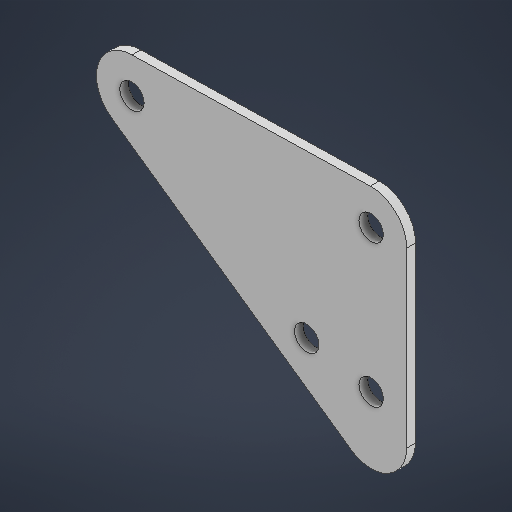
# Autodesk Inventor part: Part141
Saved by Autodesk Inventor 2025.1 (Build 291241000, 241)
## iProperties
Created: 2025-01-09
Part Number: Part141
Material: Generic
Document SubType Name: Modeling
Designer: Derek Chen
Density: 1 g/cm^3
Appearance: Default
Author: Derek Chen
Autodesk Inventor part; units mm, degrees
ref_plane "YZ Plane" through (0, 0, 0) normal (1, 0, 0) x (0, 1, 0)
ref_plane "XZ Plane" through (0, 0, 0) normal (0, 1, 0) x (-1, 0, 0)
ref_plane "XY Plane" through (0, 0, 0) normal (0, 0, 1) x (1, 0, 0)
sketch "Sketch1" plane through (0, 0, 0) normal (0, 0, 1) x (1, 0, 0)
  circle A0 centre (23.9168, 13.1886) radius 2.1844
  ellipse E0 centre (12.3891, -9.6575) end of major axis (10.2047, -9.6575) minor radius 2.1844
  ellipse E1 centre (-18.832, 12.1795) end of major axis (-21.0164, 12.1795) minor radius 2.1844
  line L0 (-18.832, 18.5295) -> (23.7667, 19.5368)
  arc A1 (-18.832, 18.5295) -> (-22.4715, 6.9759) centre (-18.832, 12.1795) ccw
  arc A2 (30.2668, 13.1886) -> (23.7667, 19.5368) centre (23.9168, 13.1886) ccw
  line L1 (-22.4715, 6.9759) -> (20.8933, -23.3546)
  line L2 (30.2668, 13.1886) -> (30.2458, -17.7636)
  arc A3 (20.8933, -23.3546) -> (30.2458, -17.7636) centre (23.8958, -17.7593) ccw
  circle A4 centre (23.9168, -12.2114) radius 2.1844
  point P0 (0, 0)
  dimension "d6" = 4.3688
  constraints: 6 end point, 6 point on circle, 5 centre point, 2 coincident, 4 other
  measures "d6" diameter of A4
extrude "Extrusion2" add sketch "Sketch1" along normal blind 1.5875
body "Solid2"
